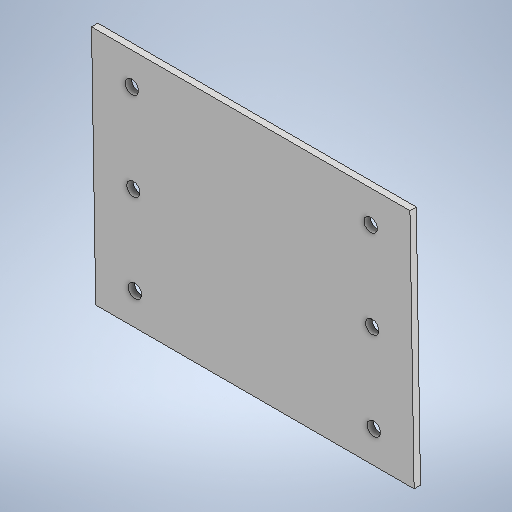
# Autodesk Inventor part: Сrane plate 3
Saved by Autodesk Inventor 2025 (Build 290162010, 162A)
## iProperties
Created: 2024-06-15
Part Number: Сrane plate 3
Material: Generic
Document SubType Name: Sheet Metal
Designer: admin
Density: 1 g/cm^3
Sheet Metal Rule: Default
Appearance: Default
Stock Number: Кран плата 3
Flat Pattern Width: 30 cm
Flat Pattern Length: 40.5237 cm
Flat Pattern Area: 1215.71 cm^2
Sheet Metal Width: 300,000 mm
Sheet Metal Length: 405,237 mm
Sheet Metal Area: 121570,956 mm^2
Author: admin
Autodesk Inventor part; units mm, degrees
ref_plane "YZ Plane" through (0, 0, 0) normal (1, 0, 0) x (0, 1, 0)
ref_plane "XZ Plane" through (0, 0, 0) normal (0, 1, 0) x (-1, 0, 0)
ref_plane "XY Plane" through (0, 0, 0) normal (0, 0, 1) x (1, 0, 0)
sketch "Sketch5" plane through (0, 0, 0) normal (0, 1, 0) x (-1, 0, 0)
  line L0 (200, 0) -> (-200, 0)
  line L1 (-205.2365, -300) -> (194.7635, -300)
  line L2 (194.7635, -300) -> (200, 0)
  line L3 (-200, 0) -> (-205.2365, -300)
  line L4 (-200, 0) -> (-200, -300) construction
  line L5 (-150.6906, -40) -> (-154.5307, -260) construction
  line L6 (149.2942, -40) -> (145.4541, -260) construction
  line L7 (145.4541, -260) -> (195.4465, -260.8726) construction
  line L8 (-154.5307, -260) -> (-204.5231, -259.1274) construction
  circle A0 centre (149.2942, -40) radius 8.5
  circle A1 centre (147.3741, -150) radius 8.5
  circle A2 centre (145.4541, -260) radius 8.5
  circle A3 centre (-150.6906, -40) radius 8.5
  circle A4 centre (-152.6106, -150) radius 8.5
  circle A5 centre (-154.5307, -260) radius 8.5
  point P0 (0, 0)
  point P1 (0, 0)
  dimension "d26" = 400
  dimension "d27" = 1
  dimension "d28" = 400
  dimension "d29" = 300
  dimension "d31" = 50
  dimension "d33" = 40
  dimension "d34" = 40
  dimension "d35" = 17
  measures "d26" distance of L0.start L0.end
  measures "d27" angle of L4 L3
  measures "d28" distance of L1.start L1.end
  measures "d29" distance between parallel lines of L1 L0
  measures "d31" distance between parallel lines of L2 L6
  measures "d33" distance from line of L0 L6.start
  measures "d34" distance from line of L1 L6.end
  measures "d35" diameter of A0
extrude "Plate3" add sketch "Sketch5" along normal blind 8
equation "\"d28\" = d26"
equation "\"d34\" = d33"
equation "\"d30\" = Thickness"
equation "\"BendRadius\" = Thickness"
equation "\"BendReliefWidth\" = Thickness"
equation "\"BendReliefDepth\" = 0.5 * Thickness"
equation "\"CornerReliefSize\" = 4 * Thickness"
equation "\"MinimumRemnant\" = 2 * Thickness"
equation "\"TransitionRadius\" = BendRadius"
equation "\"JacobiRadiusSize\" = BendRadius"
equation "\"GapSize\" = Thickness"
equation "\"Thickness\" = 8"
body "Solid2"
